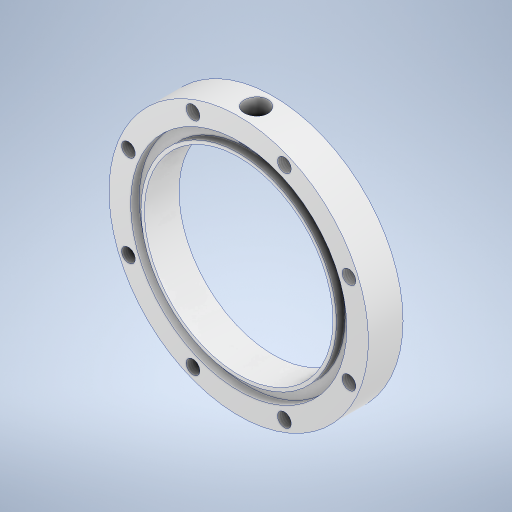
# Autodesk Inventor part: front
Saved by Autodesk Inventor 2023 (Build 270158000, 158)
## iProperties
Created: 2022-09-21
Part Number: front
Material: Aluminum 6061
Document SubType Name: Modeling
Designer: station
Density: 2.7 g/cm^3
Appearance: Aluminum - Flat
Author: station
Autodesk Inventor part; units mm, degrees
ref_plane "YZ Plane" through (0, 0, 0) normal (1, 0, 0) x (0, 1, 0)
ref_plane "XY Plane" through (0, 0, 0) normal (0, 0, 1) x (1, 0, 0)
sketch "Sketch1" plane through (0, 0, 0) normal (0, 0, 1) x (1, 0, 0)
  circle A0 centre (0, 0) radius 54.5
  circle A1 centre (0, 0) radius 75
  circle A2 centre (0, 0) radius 56.5
  circle A3 centre (0, 0) radius 62.5
  circle A4 centre (0, 0) radius 69
  line L0 (0, 0) -> (0, 69) construction
  line L1 (0, 0) -> (26.4052, 63.7477) construction
  line L2 (0, 0) -> (69, 0) construction
  circle A5 centre (26.4052, 63.7477) radius 4
  dimension "d0" = 109
  dimension "d1" = 150
  dimension "d2" = 113
  dimension "d3" = 125
  dimension "d4" = 138
  dimension "d16" = 67.5
  dimension "d17" = 8
  constraints: 6 centre point, 6 coincident, 6 end point, 2 point on circle, 1 equal length, 1 horizontal, 1 vertical
  measures "d0" diameter of A0
  measures "d1" diameter of A1
  measures "d2" diameter of A2
  measures "d3" diameter of A3
  measures "d4" diameter of A4
  measures "d16" angle of L2 L1
  measures "d17" diameter of A5
extrude "Extrusion1" add sketch "Sketch1" along normal blind 20 contours A2
extrude "Extrusion2" add sketch "Sketch1" along normal blind 15 contours A3
extrude "Extrusion3" add sketch "Sketch1" along normal blind 20 contours A1 | A4 A5 | A5 A4 | A4 A5
ref_plane "Work Plane1" through (0, 75, 0) normal (0, 1, 0) x (-1, 0, 0)
sketch "Sketch2" plane through (0, 75, 0) normal (0, 1, 0) x (-1, 0, 0)
  line L0 (0, 0) -> (0, 10) construction
  circle A0 centre (0, 10) radius 6.858
  dimension "d12" = 10
  dimension "d13" = 13.716
  constraints: 2 end point, 1 centre point, 1 coincident, 1 vertical
  measures "d12" distance of L0.start L0.end
  measures "d13" diameter of A0
extrude "Extrusion4" cut sketch "Sketch2" against normal blind 18
extrude "Extrusion5" cut sketch "Sketch1" along normal through all contours A5 A4 | A4 A5 picked at (25.7495, 62.5769) picked at (26.9375, 64.9608)
thread "Thread2" size "M8x1.25" class "6H" standard "ANSI Metric M Profile" full length
pattern_circular "Circular Pattern2" count 8 over 360 about axis through (0, 0, -10) along (0, 0, 1) of "Extrusion5"
thread "Thread13" size "M8x1.25" class "6H" standard "ANSI Metric M Profile" full length
thread "Thread14" size "M8x1.25" class "6H" standard "ANSI Metric M Profile" full length
thread "Thread15" size "M8x1.25" class "6H" standard "ANSI Metric M Profile" full length
thread "Thread16" size "M8x1.25" class "6H" standard "ANSI Metric M Profile" full length
thread "Thread17" size "M8x1.25" class "6H" standard "ANSI Metric M Profile" full length
thread "Thread18" size "M8x1.25" class "6H" standard "ANSI Metric M Profile" full length
thread "Thread19" size "M8x1.25" class "6H" standard "ANSI Metric M Profile" full length
thread "Thread20" size "M8x1.25" class "6H" standard "ANSI Metric M Profile" full length
body "Solid1"
